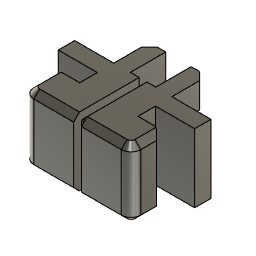
Switch_Slide v5 (Autodesk Fusion 360 design; units mm, degrees)
Autodesk Fusion 360 part; units mm, degrees
sketch "Sketch1" plane through (0, -3.8, 0) normal (0, -1, 0) x (1, 0, 0)
  line L0 (7.2432, -2.0207) -> (7.2432, -6.0207)
  line L1 (7.2432, -6.0207) -> (6.5829, -6.0207)
  line L2 (6.5829, -6.0207) -> (6.5829, -2.0207)
  line L3 (6.5829, -2.0207) -> (7.2432, -2.0207)
  line L4 (18.9458, -2.6974) -> (18.9458, -6.0207)
  line L5 (18.9458, -6.0207) -> (18.2855, -6.0207)
  line L6 (18.2855, -6.0207) -> (18.2855, -2.6974)
  line L7 (18.2855, -2.6974) -> (17.3114, -2.6974)
  line L8 (17.3114, -2.6974) -> (17.3114, -2.0207)
  line L9 (17.3114, -2.0207) -> (19.9171, -2.0207)
  line L10 (19.9171, -2.0207) -> (19.9171, -2.6974)
  line L11 (19.9171, -2.6974) -> (18.9458, -2.6974)
  spline S0 degree 3 poles (14.3632, -5.3863) (14.3259, -5.2286) (14.2301, -4.8244) (14.2323, -4.4082) (14.2336, -4.1544) knots 0 0 0 0 0.048494 0.124246 0.124246 0.124246 0.124246
  line L12 (14.2336, -4.1544) -> (14.2336, -2.0207)
  line L13 (14.2336, -2.0207) -> (14.8939, -2.0207)
  line L14 (14.8939, -2.0207) -> (14.8939, -4.1872)
  spline S1 degree 3 poles (14.8939, -4.1872) (14.8933, -4.3262) (14.8922, -4.5458) (14.9115, -4.7645) (14.9185, -4.8447) knots 0 0 0 0 0.041683 0.065832 0.065832 0.065832 0.065832
  spline S2 degree 3 poles (14.9185, -4.8447) (14.9365, -4.9265) (14.9707, -5.0815) (15.0773, -5.1986) (15.1277, -5.254) knots 0 0 0 0 0.024609 0.046682 0.046682 0.046682 0.046682
  spline S3 degree 3 poles (15.1277, -5.254) (15.1896, -5.2961) (15.3208, -5.3855) (15.4798, -5.3941) (15.5638, -5.3986) knots 0 0 0 0 0.02203 0.046732 0.046732 0.046732 0.046732
  spline S4 degree 3 poles (15.5638, -5.3986) (15.6349, -5.3957) (15.7679, -5.3901) (15.8842, -5.3261) (15.9384, -5.2963) knots 0 0 0 0 0.021004 0.039303 0.039303 0.039303 0.039303
  spline S5 degree 3 poles (15.9384, -5.2963) (15.9831, -5.2584) (16.0739, -5.1812) (16.1155, -5.0694) (16.1367, -5.0125) knots 0 0 0 0 0.017262 0.035135 0.035135 0.035135 0.035135
  spline S6 degree 3 poles (16.1367, -5.0125) (16.152, -4.9175) (16.1935, -4.6599) (16.1913, -4.3985) (16.19, -4.2335) knots 0 0 0 0 0.028826 0.078196 0.078196 0.078196 0.078196
  line L15 (16.19, -4.2335) -> (16.19, -2.0207)
  line L16 (16.19, -2.0207) -> (16.8503, -2.0207)
  line L17 (16.8503, -2.0207) -> (16.8503, -4.1217)
  spline S7 degree 3 poles (16.8503, -4.1217) (16.8503, -4.3534) (16.8504, -4.7437) (16.7892, -5.1289) (16.7643, -5.2854) knots 0 0 0 0 0.069372 0.116844 0.116844 0.116844 0.116844
  spline S8 degree 3 poles (16.7643, -5.2854) (16.7265, -5.3995) (16.6505, -5.6286) (16.4683, -5.787) (16.3769, -5.8666) knots 0 0 0 0 0.035352 0.071003 0.071003 0.071003 0.071003
  spline S9 degree 3 poles (16.3769, -5.8666) (16.263, -5.9313) (16.0171, -6.0712) (15.7337, -6.0827) (15.5815, -6.0889) knots 0 0 0 0 0.038734 0.083656 0.083656 0.083656 0.083656
  spline S10 degree 3 poles (15.5815, -6.0889) (15.4265, -6.0851) (15.1461, -6.0782) (14.8936, -5.9583) (14.7807, -5.9048) knots 0 0 0 0 0.0459 0.082982 0.082982 0.082982 0.082982
  spline S11 degree 3 poles (14.7807, -5.9048) (14.6911, -5.8364) (14.5095, -5.6979) (14.4124, -5.4911) (14.3632, -5.3863) knots 0 0 0 0 0.033286 0.067442 0.067442 0.067442 0.067442
  spline S12 degree 3 poles (41.3039, -5.3863) (41.2665, -5.2286) (41.1708, -4.8244) (41.1729, -4.4082) (41.1743, -4.1544) knots 0 0 0 0 0.048494 0.124246 0.124246 0.124246 0.124246
  line L18 (41.1743, -4.1544) -> (41.1743, -2.0207)
  line L19 (41.1743, -2.0207) -> (41.8346, -2.0207)
  line L20 (41.8346, -2.0207) -> (41.8346, -4.1872)
  spline S13 degree 3 poles (41.8346, -4.1872) (41.8339, -4.3262) (41.8329, -4.5458) (41.8521, -4.7645) (41.8592, -4.8447) knots 0 0 0 0 0.041682 0.065832 0.065832 0.065832 0.065832
  spline S14 degree 3 poles (41.8592, -4.8447) (41.8772, -4.9265) (41.9114, -5.0815) (42.018, -5.1986) (42.0684, -5.254) knots 0 0 0 0 0.024609 0.046683 0.046683 0.046683 0.046683
  spline S15 degree 3 poles (42.0684, -5.254) (42.1302, -5.2961) (42.2614, -5.3855) (42.4204, -5.3941) (42.5045, -5.3986) knots 0 0 0 0 0.02203 0.046732 0.046732 0.046732 0.046732
  spline S16 degree 3 poles (42.5045, -5.3986) (42.5756, -5.3957) (42.7086, -5.3901) (42.8249, -5.3261) (42.8791, -5.2963) knots 0 0 0 0 0.021004 0.039303 0.039303 0.039303 0.039303
  spline S17 degree 3 poles (42.8791, -5.2963) (42.9237, -5.2584) (43.0146, -5.1812) (43.0562, -5.0694) (43.0773, -5.0125) knots 0 0 0 0 0.017262 0.035135 0.035135 0.035135 0.035135
  spline S18 degree 3 poles (43.0773, -5.0125) (43.0926, -4.9175) (43.1341, -4.6599) (43.132, -4.3985) (43.1306, -4.2335) knots 0 0 0 0 0.028826 0.078196 0.078196 0.078196 0.078196
  line L21 (43.1306, -4.2335) -> (43.1306, -2.0207)
  line L22 (43.1306, -2.0207) -> (43.7909, -2.0207)
  line L23 (43.7909, -2.0207) -> (43.7909, -4.1217)
  spline S19 degree 3 poles (43.7909, -4.1217) (43.791, -4.3534) (43.791, -4.7437) (43.7298, -5.1289) (43.705, -5.2854) knots 0 0 0 0 0.069372 0.116844 0.116844 0.116844 0.116844
  spline S20 degree 3 poles (43.705, -5.2854) (43.6671, -5.3995) (43.5911, -5.6286) (43.409, -5.787) (43.3175, -5.8666) knots 0 0 0 0 0.035352 0.071003 0.071003 0.071003 0.071003
  spline S21 degree 3 poles (43.3175, -5.8666) (43.2037, -5.9313) (42.9578, -6.0712) (42.6744, -6.0827) (42.5222, -6.0889) knots 0 0 0 0 0.038734 0.083656 0.083656 0.083656 0.083656
  spline S22 degree 3 poles (42.5222, -6.0889) (42.3671, -6.0851) (42.0868, -6.0782) (41.8342, -5.9583) (41.7214, -5.9048) knots 0 0 0 0 0.0459 0.082982 0.082982 0.082982 0.082982
  spline S23 degree 3 poles (41.7214, -5.9048) (41.6317, -5.8364) (41.4501, -5.6979) (41.3531, -5.4911) (41.3039, -5.3863) knots 0 0 0 0 0.033286 0.067442 0.067442 0.067442 0.067442
  spline S24 degree 3 poles (50.4662, -5.3863) (50.4289, -5.2286) (50.3331, -4.8244) (50.3353, -4.4082) (50.3366, -4.1544) knots 0 0 0 0 0.048494 0.124246 0.124246 0.124246 0.124246
  line L24 (50.3366, -4.1544) -> (50.3366, -2.0207)
  line L25 (50.3366, -2.0207) -> (50.9969, -2.0207)
  line L26 (50.9969, -2.0207) -> (50.9969, -4.1872)
  spline S25 degree 3 poles (50.9969, -4.1872) (50.9963, -4.3262) (50.9952, -4.5458) (51.0145, -4.7645) (51.0215, -4.8447) knots 0 0 0 0 0.041682 0.065832 0.065832 0.065832 0.065832
  spline S26 degree 3 poles (51.0215, -4.8447) (51.0395, -4.9265) (51.0737, -5.0815) (51.1803, -5.1986) (51.2307, -5.254) knots 0 0 0 0 0.024609 0.046683 0.046683 0.046683 0.046683
  spline S27 degree 3 poles (51.2307, -5.254) (51.2926, -5.2961) (51.4238, -5.3855) (51.5828, -5.3941) (51.6668, -5.3986) knots 0 0 0 0 0.022029 0.046732 0.046732 0.046732 0.046732
  spline S28 degree 3 poles (51.6668, -5.3986) (51.7379, -5.3957) (51.8709, -5.3901) (51.9872, -5.3261) (52.0414, -5.2963) knots 0 0 0 0 0.021004 0.039303 0.039303 0.039303 0.039303
  spline S29 degree 3 poles (52.0414, -5.2963) (52.0861, -5.2584) (52.1769, -5.1812) (52.2185, -5.0694) (52.2397, -5.0125) knots 0 0 0 0 0.017262 0.035135 0.035135 0.035135 0.035135
  spline S30 degree 3 poles (52.2397, -5.0125) (52.255, -4.9175) (52.2965, -4.6599) (52.2943, -4.3985) (52.293, -4.2335) knots 0 0 0 0 0.028826 0.078196 0.078196 0.078196 0.078196
  line L27 (52.293, -4.2335) -> (52.293, -2.0207)
  line L28 (52.293, -2.0207) -> (52.9533, -2.0207)
  line L29 (52.9533, -2.0207) -> (52.9533, -4.1217)
  spline S31 degree 3 poles (52.9533, -4.1217) (52.9533, -4.3534) (52.9534, -4.7437) (52.8922, -5.1289) (52.8673, -5.2854) knots 0 0 0 0 0.069372 0.116844 0.116844 0.116844 0.116844
  spline S32 degree 3 poles (52.8673, -5.2854) (52.8295, -5.3995) (52.7535, -5.6286) (52.5713, -5.787) (52.4799, -5.8666) knots 0 0 0 0 0.035352 0.071003 0.071003 0.071003 0.071003
  spline S33 degree 3 poles (52.4799, -5.8666) (52.366, -5.9313) (52.1201, -6.0712) (51.8367, -6.0827) (51.6845, -6.0889) knots 0 0 0 0 0.038734 0.083656 0.083656 0.083656 0.083656
  spline S34 degree 3 poles (51.6845, -6.0889) (51.5295, -6.0851) (51.2491, -6.0782) (50.9966, -5.9583) (50.8837, -5.9048) knots 0 0 0 0 0.0459 0.082982 0.082982 0.082982 0.082982
  spline S35 degree 3 poles (50.8837, -5.9048) (50.7941, -5.8364) (50.6125, -5.6979) (50.5154, -5.4911) (50.4662, -5.3863) knots 0 0 0 0 0.033286 0.067442 0.067442 0.067442 0.067442
  line L30 (47.9465, -4.5119) -> (47.9465, -6.0207)
  line L31 (47.9465, -6.0207) -> (47.2862, -6.0207)
  line L32 (47.2862, -6.0207) -> (47.2862, -2.0207)
  line L33 (47.2862, -2.0207) -> (48.3503, -2.0207)
  spline S36 degree 3 poles (48.3503, -2.0207) (48.5148, -2.0193) (48.7759, -2.0171) (49.0328, -2.0616) (49.1279, -2.078) knots 0 0 0 0 0.049202 0.078105 0.078105 0.078105 0.078105
  spline S37 degree 3 poles (49.1279, -2.078) (49.2222, -2.1197) (49.419, -2.2067) (49.5442, -2.3822) (49.6095, -2.4737) knots 0 0 0 0 0.030342 0.063355 0.063355 0.063355 0.063355
  spline S38 degree 3 poles (49.6095, -2.4737) (49.6647, -2.5872) (49.7843, -2.833) (49.7939, -3.1067) (49.7991, -3.254) knots 0 0 0 0 0.037457 0.081099 0.081099 0.081099 0.081099
  spline S39 degree 3 poles (49.7991, -3.254) (49.7943, -3.389) (49.7853, -3.642) (49.6831, -3.8733) (49.6354, -3.9812) knots 0 0 0 0 0.04008 0.075144 0.075144 0.075144 0.075144
  spline S40 degree 3 poles (49.6354, -3.9812) (49.5799, -4.0704) (49.4749, -4.2394) (49.3059, -4.3438) (49.2261, -4.3932) knots 0 0 0 0 0.031024 0.058778 0.058778 0.058778 0.058778
  spline S41 degree 3 poles (49.2261, -4.3932) (49.1155, -4.4275) (48.8408, -4.5126) (48.5525, -4.5121) (48.3803, -4.5119) knots 0 0 0 0 0.034589 0.085835 0.085835 0.085835 0.085835
  line L34 (48.3803, -4.5119) -> (47.9465, -4.5119)
  line L35 (45.8864, -2.6974) -> (45.8864, -6.0207)
  line L36 (45.8864, -6.0207) -> (45.2261, -6.0207)
  line L37 (45.2261, -6.0207) -> (45.2261, -2.6974)
  line L38 (45.2261, -2.6974) -> (44.252, -2.6974)
  line L39 (44.252, -2.6974) -> (44.252, -2.0207)
  line L40 (44.252, -2.0207) -> (46.8578, -2.0207)
  line L41 (46.8578, -2.0207) -> (46.8578, -2.6974)
  line L42 (46.8578, -2.6974) -> (45.8864, -2.6974)
  spline S42 degree 3 poles (39.0733, -6.0889) (38.8506, -6.0709) (38.4179, -6.0358) (38.1023, -5.7391) (37.9492, -5.5951) knots 0 0 0 0 0.064896 0.126084 0.126084 0.126084 0.126084
  spline S43 degree 3 poles (37.9492, -5.5951) (37.8125, -5.3779) (37.5156, -4.9061) (37.4924, -4.3471) (37.4799, -4.0453) knots 0 0 0 0 0.07567 0.164443 0.164443 0.164443 0.164443
  spline S44 degree 3 poles (37.4799, -4.0453) (37.4852, -3.8257) (37.4949, -3.4217) (37.6298, -3.0415) (37.6913, -2.8679) knots 0 0 0 0 0.065391 0.12029 0.12029 0.12029 0.12029
  spline S45 degree 3 poles (37.6913, -2.8679) (37.7636, -2.7261) (37.9004, -2.4578) (38.1338, -2.2683) (38.2439, -2.179) knots 0 0 0 0 0.047145 0.089188 0.089188 0.089188 0.089188
  spline S46 degree 3 poles (38.2439, -2.179) (38.367, -2.113) (38.6249, -1.9746) (38.9176, -1.9601) (39.0706, -1.9525) knots 0 0 0 0 0.041369 0.086677 0.086677 0.086677 0.086677
  spline S47 degree 3 poles (39.0706, -1.9525) (39.2942, -1.9746) (39.74, -2.0188) (40.0589, -2.3333) (40.2179, -2.49) knots 0 0 0 0 0.065279 0.130173 0.130173 0.130173 0.130173
  spline S48 degree 3 poles (40.2179, -2.49) (40.347, -2.7016) (40.6323, -3.1695) (40.651, -3.7194) (40.6613, -4.0207) knots 0 0 0 0 0.07314 0.161762 0.161762 0.161762 0.161762
  spline S49 degree 3 poles (40.6613, -4.0207) (40.6493, -4.3274) (40.6272, -4.8927) (40.3286, -5.3708) (40.192, -5.5896) knots 0 0 0 0 0.090193 0.166286 0.166286 0.166286 0.166286
  spline S50 degree 3 poles (40.192, -5.5896) (40.0396, -5.7352) (39.7267, -6.034) (39.2948, -6.0703) (39.0733, -6.0889) knots 0 0 0 0 0.061329 0.125849 0.125849 0.125849 0.125849
  line L43 (11.8435, -4.5119) -> (11.8435, -6.0207)
  line L44 (11.8435, -6.0207) -> (11.1832, -6.0207)
  line L45 (11.1832, -6.0207) -> (11.1832, -2.0207)
  line L46 (11.1832, -2.0207) -> (12.2473, -2.0207)
  spline S51 degree 3 poles (12.2473, -2.0207) (12.4118, -2.0193) (12.6729, -2.0171) (12.9298, -2.0616) (13.0249, -2.078) knots 0 0 0 0 0.049202 0.078105 0.078105 0.078105 0.078105
  spline S52 degree 3 poles (13.0249, -2.078) (13.1192, -2.1197) (13.316, -2.2067) (13.4412, -2.3822) (13.5065, -2.4737) knots 0 0 0 0 0.030342 0.063355 0.063355 0.063355 0.063355
  spline S53 degree 3 poles (13.5065, -2.4737) (13.5617, -2.5872) (13.6813, -2.8329) (13.6909, -3.1067) (13.6961, -3.254) knots 0 0 0 0 0.037457 0.081099 0.081099 0.081099 0.081099
  spline S54 degree 3 poles (13.6961, -3.254) (13.6913, -3.389) (13.6823, -3.642) (13.5801, -3.8733) (13.5324, -3.9812) knots 0 0 0 0 0.04008 0.075144 0.075144 0.075144 0.075144
  spline S55 degree 3 poles (13.5324, -3.9812) (13.4769, -4.0704) (13.3719, -4.2394) (13.2029, -4.3438) (13.1231, -4.3932) knots 0 0 0 0 0.031024 0.058778 0.058778 0.058778 0.058778
  spline S56 degree 3 poles (13.1231, -4.3932) (13.0125, -4.4275) (12.7378, -4.5126) (12.4494, -4.5121) (12.2773, -4.5119) knots 0 0 0 0 0.034589 0.085835 0.085835 0.085835 0.085835
  line L47 (12.2773, -4.5119) -> (11.8435, -4.5119)
  line L48 (8.501, -3.4123) -> (8.501, -6.0207)
  line L49 (8.501, -6.0207) -> (7.8844, -6.0207)
  line L50 (7.8844, -6.0207) -> (7.8844, -2.0207)
  line L51 (7.8844, -2.0207) -> (8.5283, -2.0207)
  line L52 (8.5283, -2.0207) -> (9.8707, -4.6919)
  line L53 (9.8707, -4.6919) -> (9.8707, -2.0207)
  line L54 (9.8707, -2.0207) -> (10.4874, -2.0207)
  line L55 (10.4874, -2.0207) -> (10.4874, -6.0207)
  line L56 (10.4874, -6.0207) -> (9.8216, -6.0207)
  line L57 (9.8216, -6.0207) -> (8.501, -3.4123)
  line L58 (41.75, 4.11) -> (18.25, 4.11) construction
  arc A0 (8.25, 4.11) -> (18.25, 4.11) centre (13.25, 4.11) ccw
  line L59 (8.25, 4.11) -> (2.75, 4.11)
  line L60 (2.75, 4.11) -> (2.75, -7.2897)
  line L61 (2.75, -7.2897) -> (57.25, -7.2897)
  line L62 (57.25, -7.2897) -> (57.25, 4.11)
  line L63 (56.0201, -2.6974) -> (55.0488, -2.6974)
  line L64 (55.0488, -2.6974) -> (55.0488, -6.0207)
  line L65 (55.0488, -6.0207) -> (54.3885, -6.0207)
  line L66 (54.3885, -6.0207) -> (54.3885, -2.6974)
  line L67 (54.3885, -2.6974) -> (53.4144, -2.6974)
  line L68 (53.4144, -2.6974) -> (53.4144, -2.0207)
  line L69 (53.4144, -2.0207) -> (56.0201, -2.0207)
  line L70 (57.25, 4.11) -> (51.75, 4.11)
  arc A1 (41.75, 4.11) -> (51.75, 4.11) centre (46.75, 4.11) ccw
  line L71 (25.61, 3.2758) -> (25.61, 5.2758) construction
  line L72 (25.61, 5.2758) -> (25.61, 3.2758) construction
  line L73 (27.61, 5.2758) -> (25.61, 5.2758) construction
  line L74 (25.61, 5.2758) -> (26.0414, 5.2758) construction
  line L75 (26.0414, 5.2758) -> (26.61, 5.2758) construction
  line L76 (26.61, 5.2758) -> (27.1786, 5.2758) construction
  line L77 (27.1786, 5.2758) -> (27.61, 5.2758) construction
  line L78 (27.61, 3.2758) -> (27.61, 5.2758)
  line L79 (27.61, 5.2758) -> (27.61, 3.2758)
  line L80 (25.61, 3.2758) -> (27.61, 3.2758) construction
  line L81 (25.61, 5.2758) -> (27.61, 3.2758) construction
  line L82 (25.61, 3.2758) -> (27.61, 5.2758) construction
  line L83 (26.61, 4.2758) -> (28.61, 4.2758) construction
  line L84 (29.61, 3.2758) -> (27.61, 3.2758)
  line L85 (27.61, 3.2758) -> (27.61, 5.2758)
  line L86 (27.61, 5.2758) -> (29.61, 5.2758)
  line L87 (29.61, 5.2758) -> (29.61, 3.2758)
  line L88 (29.61, 3.2758) -> (27.61, 5.2758) construction
  line L89 (27.61, 3.2758) -> (29.61, 5.2758) construction
  line L90 (27.31, 2.9758) -> (27.31, 5.5758)
  line L91 (27.31, 5.5758) -> (29.91, 5.5758)
  line L92 (29.91, 5.5758) -> (29.91, 2.9758)
  line L93 (29.91, 2.9758) -> (27.31, 2.9758)
  line L94 (29.91, 5.5758) -> (31.58, 5.5758)
  line L95 (31.58, 5.5758) -> (31.58, 2.9758)
  line L96 (31.58, 2.9758) -> (29.91, 2.9758)
  line L97 (27.31, 5.5758) -> (25.64, 5.5758)
  line L98 (25.64, 5.5758) -> (25.64, 2.9758)
  line L99 (25.64, 2.9758) -> (27.31, 2.9758)
  line L100 (23.14, 5.5758) -> (34.08, 5.5758)
  line L101 (34.08, 5.5758) -> (34.08, -1.4242)
  line L102 (34.08, -1.4242) -> (23.14, -1.4242)
  line L103 (23.14, -1.4242) -> (23.14, 5.5758)
  line L104 (56.0201, -2.0207) -> (56.0201, -2.6974)
  point P0 (28.61, 4.2758)
  dimension "d340" = 2
  dimension "d345" = -0.3
  dimension "d346" = 1.67
  dimension "d347" = 1.67
  dimension "d365" = 2.5
  dimension "d366" = 2.5
  dimension "d367" = 7
  constraint coincident L71.start L72.end
  constraint coincident L78.start L79.end
  constraint coincident L71.end L72.start
  constraint coincident L73.start L77.end
  constraint midpoint L81 L83.start
  constraint perpendicular L78 L83
  constraint horizontal L84
  constraint perpendicular L84 L85
  constraint parallel L84 L86
  constraint parallel L85 L87
  constraint coincident L88 P0
  constraint coincident L89 P0
  constraint coincident P0 L83.end
  constraint equal L71 L85
  constraint equal L80 L84
  constraint perpendicular L92 L94
  constraint perpendicular L93 L95
  constraint perpendicular L92 L96
  constraint perpendicular L90 L97
  constraint perpendicular L93 L98
  constraint perpendicular L90 L99
  constraint horizontal L100
  constraint vertical L101
  constraint horizontal L102
  constraint vertical L103
  constraint coincident L97.end L100
  measures "d340" distance of L83.start P0
  measures "d346" distance of L91.end L94.end
  measures "d347" distance of L90.start L98.end
  measures "d365" distance of L95 L101
  measures "d366" distance of L98 L103
  measures "d367" distance of L100 L102
extrude "Extrude1" add sketch "Sketch1" against normal blind 7.115 contours L90 L97 L98 L99 L100 | L92 L94 L95 L96 L100 makes body 1 at (29.91, -1.4283, 4.7091) makes body 2 at (25.64, -1.4283, 4.7091)
extrude "Extrude2" add sketch "Sketch1" along normal blind 3.2 contours L78 L79 L84 L85 L86 L87 | L90 L97 L98 L99 L100 | L90 L91 L92 L93 L100 | L93 L95 L96 L98 L99 L100 L101 L102 L103 | L92 L94 L95 L96 L100 bodies 1 2
sketch "Catch" plane through (0, 0, 5.5758) normal (0, 0, 1) x (-1, 0, 0)
  line L0 (-34.08, 7) -> (-34.08, 3.8)
  line L1 (-34.08, 3.8) -> (-31.58, 3.8)
  line L2 (-31.58, 3.8) -> (-31.58, -3.3151)
  line L3 (-31.58, -3.3151) -> (-29.91, -3.3151)
  line L4 (-29.91, -3.3151) -> (-29.91, 3.8)
  line L5 (-29.91, 3.8) -> (-27.31, 3.8)
  line L6 (-27.31, 3.8) -> (-27.31, -3.3151)
  line L7 (-27.31, -3.3151) -> (-25.64, -3.3151)
  line L8 (-25.64, -3.3151) -> (-25.64, 3.8)
  line L9 (-25.64, 3.8) -> (-23.14, 3.8)
  line L10 (-23.14, 3.8) -> (-23.14, 7)
  line L11 (-23.14, 7) -> (-34.08, 7)
  line L12 (-31.58, 2) -> (-35.58, 2)
  line L13 (-35.58, 2) -> (-35.58, 0.33)
  line L14 (-35.58, 0.33) -> (-31.58, 0.33)
  line L15 (-25.64, 0.33) -> (-21.64, 0.33)
  line L16 (-21.64, 0.33) -> (-21.64, 2)
  line L17 (-21.64, 2) -> (-25.64, 2)
  line L18 (-25.64, 2) -> (-31.58, 2)
  line L19 (-40.2186, 2.2) -> (-19.7814, 2.2)
  line L20 (-25.64, 0.33) -> (-31.58, 0.33)
  dimension "d354" = 0.2
  dimension "d355" = 1.67
  dimension "d356" = 4
  dimension "d357" = 4
  constraint coincident L2 L12.start
  constraint perpendicular L2 L12
  constraint perpendicular L12 L13
  constraint coincident L2 L14.end
  constraint perpendicular L2 L14
  constraint coincident L8 L15.start
  constraint perpendicular L8 L15
  constraint perpendicular L15 L16
  constraint coincident L8 L17.end
  constraint perpendicular L8 L17
  constraint horizontal L18
  constraint horizontal L20
  measures "d354" distance of L12 L19
  measures "d355" distance of L12 L14
  measures "d356" distance of L8 L16
  measures "d357" distance of L2 L13
extrude "Extrude3" add sketch "Catch" against normal up to surface (7 mm away) contours L2 L4 L18 L20 | L2 L12 L13 L14 | L4 L6 L18 L20 | L8 L15 L16 L17 | L6 L8 L18 L20 bodies 1
extrude "Extrude4" add sketch "Sketch1" against normal blind 3.5 contours L78 L79 L84 L85 L86 L87 | L90 L91 L92 L93 L100 bodies 1
fillet "Fillet1" radius 1 2 edges at (23.14, -7, 2.0758) (34.08, -7, 2.0758) on bodies 1
chamfer "Chamfer3" distance 0.6 angle 45 10 edges at (28.61, -7, 5.5758) (23.4329, -6.7071, 5.5758) (23.14, -4.9, 5.5758) (34.08, -4.9, 5.5758) (33.7871, -6.7071, 5.5758) (28.61, -7, -1.4242) (33.7871, -6.7071, -1.4242) (34.08, -4.9, -1.4242) (23.14, -4.9, -1.4242) (23.4329, -6.7071, -1.4242) on bodies 1
sketch "Cutout" plane through (0, -3.8, 0) normal (0, -1, 0) x (1, 0, 0)
  line L0 (44.0236, 8.3013) -> (15.9764, 8.3013)
  arc A0 (18.25, 4.11) -> (15.9764, 8.3013) centre (13.25, 4.11) ccw
  line L1 (18.25, 4.11) -> (41.75, 4.11) construction
  arc A1 (44.0236, 8.3013) -> (41.75, 4.11) centre (46.75, 4.11) ccw
  line L2 (25.64, 5.5758) -> (25.64, 2.9758)
  line L3 (23.14, 5.5758) -> (34.08, 5.5758) construction
  line L4 (25.64, 2.9758) -> (27.31, 2.9758)
  line L5 (29.91, 2.9758) -> (27.31, 2.9758)
  line L6 (31.58, 2.9758) -> (29.91, 2.9758)
  line L7 (31.58, 5.5758) -> (31.58, 2.9758)
  line L8 (25.64, 5.5758) -> (31.58, 2.9758) construction
  line L9 (25.64, 2.9758) -> (31.58, 5.5758) construction
  line L10 (25.64, 5.5758) -> (31.58, 5.5758) construction
  line L11 (31.58, 5.5758) -> (31.58, 2.9758) construction
  line L12 (31.58, 2.9758) -> (25.64, 2.9758) construction
  line L13 (25.64, 2.9758) -> (25.64, 5.5758) construction
  line L14 (23.64, 5.5758) -> (29.58, 5.5758) construction
  line L15 (29.58, 5.5758) -> (29.58, 2.9758) construction
  line L16 (29.58, 2.9758) -> (23.64, 2.9758) construction
  line L17 (23.64, 2.9758) -> (23.64, 5.5758) construction
  line L18 (29.58, 2.9758) -> (23.64, 5.5758) construction
  line L19 (23.64, 2.9758) -> (29.58, 5.5758) construction
  line L20 (26.61, 4.2758) -> (28.61, 4.2758) construction
  line L21 (23.34, 5.7258) -> (31.88, 5.7258)
  line L22 (31.88, 5.7258) -> (31.88, 2.8258)
  line L23 (31.88, 2.8258) -> (23.34, 2.8258)
  line L24 (23.34, 2.8258) -> (23.34, 5.7258)
  dimension "d369" = 2
  dimension "d370" = 0.3
  dimension "d371" = 0.15
  dimension "d372" = 0.15
  dimension "d373" = 0.3
  constraint coincident L2.start L8.start
  constraint coincident L6.start L7.end
  constraint coincident L2.end L4.start
  constraint coincident L7.start L9.end
  constraint horizontal L10
  constraint vertical L11
  constraint horizontal L12
  constraint vertical L13
  constraint horizontal L14
  constraint vertical L15
  constraint horizontal L16
  constraint vertical L17
  constraint coincident L12 L15.end
  constraint coincident L3 L14.start
  constraint equal L12 L16
  constraint midpoint L19 L20.start
  constraint midpoint L9 L20.end
  constraint horizontal L21
  constraint vertical L22
  constraint horizontal L23
  constraint vertical L24
  measures "d369" distance of L20.start L20.end
  measures "d370" distance of L17 L24
  measures "d371" distance of L14 L21
  measures "d372" distance of L16 L23
  measures "d373" distance of L11 L22
ref_plane "WorkPlane1" through (28.61, -5.4, 2.0758) normal (1, 0, 0) x (0, 0, 1)
sketch "POwerGroove" plane through (28.61, -4.9, 2.0758) normal (1, 0, 0) x (0, 1, 0)
  line L0 (4.57, -3.5) -> (4.57, 0.9)
  line L1 (4.57, 0.9) -> (4.6, 0.9)
  line L2 (4.6, 0.9) -> (4.6, 3.5)
  line L3 (4.6, 3.5) -> (-1.5, 3.5)
  line L4 (-1.5, 3.5) -> (-2.1, 2.9)
  line L5 (-2.1, 2.9) -> (-2.1, -2.9)
  line L6 (-2.1, -2.9) -> (-1.5, -3.5)
  line L7 (-1.5, -3.5) -> (1.1, -3.5)
  line L8 (1.1, -3.5) -> (1.1, 0.9)
  line L9 (2.9, 0.9) -> (2.9, -3.5)
  line L10 (2.9, -3.5) -> (4.57, -3.5)
  line L11 (-1.1686, -2.7) -> (0.3, -2.7)
  line L12 (0.3, -2.7) -> (0.3, 1.7)
  line L13 (0.3, 1.7) -> (3.7, 1.7)
  line L14 (3.7, 1.7) -> (3.7, -2.7)
  line L15 (3.7, -2.7) -> (3.77, -2.7)
  line L16 (3.77, -2.7) -> (3.77, 1.7)
  line L17 (3.77, 1.7) -> (3.8, 1.7)
  line L18 (3.8, 1.7) -> (3.8, 2.7)
  line L19 (3.8, 2.7) -> (-1.1686, 2.7)
  line L20 (-1.1686, 2.7) -> (-1.3, 2.5686)
  line L21 (-1.3, 2.5686) -> (-1.3, -2.5686)
  line L22 (-1.3, -2.5686) -> (-1.1686, -2.7)
  line L23 (3.8, 2.7) -> (4.6, 2.7)
  line L24 (0.3, -2.7) -> (1.1, -2.7)
  line L25 (1.1, 0.9) -> (2.9, 0.9)
  constraint coincident L2 L23.end
  constraint perpendicular L18 L23
  constraint coincident L8 L24.end
  constraint perpendicular L8 L24
extrude "Extrude5" cut sketch "POwerGroove" along normal mid plane 0.8 contours L2 L3 L4 L5 L6 L7 L8 L11 L19 L20 L21 L22 L23 L24 bodies 1
sketch "Sketch2" plane through (30, 20, 1.57) normal (0, 0, 1) x (1, 0, 0)
chamfer "Chamfer4" distance 0.6 angle 45 2 edges at (23.14, -3.8, 2.0758) (34.08, -3.8, 2.0758) on bodies 1
chamfer "Chamfer5" distance 0.8 angle 45 2 edges at (31.58, 3.315, 4.2758) (25.64, 3.315, 4.2758) on bodies 1
extrude "Extrude6" add 1 faces at (27.62, -2.6, 2.9758) along direction (0, 0, -1) blind 2 on bodies 1 bodies 1
fillet "Fillet2" radius 0.6 2 edges at (23.74, -3.8, 2.0758) (33.48, -3.8, 2.0758) on bodies 1
named bodies: "Switch_Slide"
